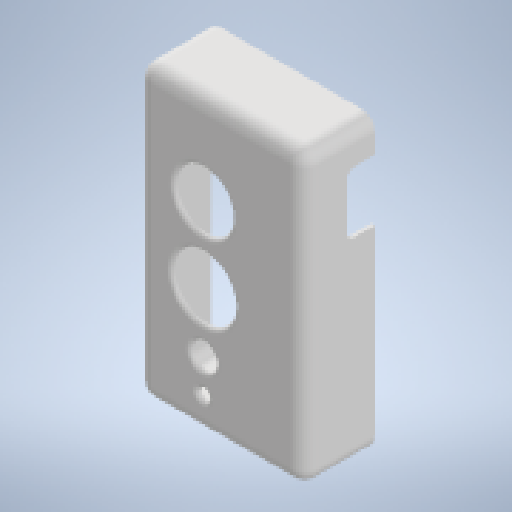
# Autodesk Inventor part: Part2
Saved by Autodesk Inventor 2025.2 (Build 292293000, 293)
## iProperties
Created: 2026-02-22
Part Number: Part2
Material: 一般
Document SubType Name: Modeling
Designer: naka6
Density: 1 g/cm^3
Appearance: 既定
Author: naka6
Autodesk Inventor part; units mm, degrees
ref_plane "YZ Plane" through (0, 0, 0) normal (1, 0, 0) x (0, 1, 0)
ref_plane "XZ Plane" through (0, 0, 0) normal (0, 1, 0) x (-1, 0, 0)
ref_plane "XY Plane" through (0, 0, 0) normal (0, 0, 1) x (1, 0, 0)
sketch "スケッチ1" plane through (0, 0, 0) normal (0, 0, 1) x (1, 0, 0)
  line L0 (17.8, -27.8) -> (17.8, 27.8) projected
  arc A0 (17.8, 27.8) -> (14.8, 30.8) centre (14.8, 27.8) ccw projected
  line L1 (14.8, 30.8) -> (-14.8, 30.8) projected
  arc A1 (-14.8, 30.8) -> (-17.8, 27.8) centre (-14.8, 27.8) ccw projected
  line L2 (-17.8, 27.8) -> (-17.8, -27.8) projected
  arc A2 (-17.8, -27.8) -> (-14.8, -30.8) centre (-14.8, -27.8) ccw projected
  line L3 (-14.8, -30.8) -> (14.8, -30.8) projected
  arc A3 (14.8, -30.8) -> (17.8, -27.8) centre (14.8, -27.8) ccw projected
  point P0 (0, 0)
extrude "押し出し1" add sketch "スケッチ1" along normal blind 15
fillet "フィレット1" radius 3 8 edges at (-16.9213, 29.9213, 15) (-17.8, 0, 15) (-16.9213, -29.9213, 15) (0, -30.8, 15) (16.9213, -29.9213, 15) (17.8, 0, 15) (16.9213, 29.9213, 15) (0, 30.8, 15)
shell "シェル1" thickness 0.8 removed faces 1 at (5.9333, 9.2667, 0)
sketch "スケッチ2" plane through (17.8, -27.8, 0) normal (1, 0, 0) x (0, 0, -1)
  line L0 (0, 51.6) -> (-6, 51.6)
  line L1 (-6, 51.6) -> (-6, 38.6)
  line L2 (-6, 38.6) -> (0, 38.6)
  line L3 (0, 38.6) -> (0, 51.6)
  line L4 (0, 58.6) -> (-12, 58.6) projected
  line L5 (0, 0) -> (0, 55.6) projected
  point P0 (0, 27.8)
  dimension "d4" = 6
  dimension "d5" = 7
  dimension "d6" = 20
  constraints: 8 end point, 2 parallel, 1 horizontal, 1 perpendicular, 1 point on line
  measures "d4" distance of L2.end L1.end
  measures "d5" distance between parallel lines of L0 L4
  measures "d6" distance between parallel lines of L4 L2
extrude "押し出し2" cut sketch "スケッチ2" against normal blind 15
fillet "フィレット2" radius 1.5 2 edges at (17.4, 10.8, 6) (17.4, 23.8, 6)
sketch "スケッチ3" plane through (0, 0, 15) normal (0, 0, 1) x (1, 0, 0)
  line L0 (-17.8, 27.8) -> (-17.8, -27.8) projected
  line L1 (-14.8, -30.8) -> (14.8, -30.8) projected
  line L2 (17.8, -27.8) -> (17.8, 27.8) projected
  line L3 (14.8, 30.8) -> (-14.8, 30.8) projected
  circle A0 centre (-3.8, 11.8) radius 6.15
  circle A1 centre (-3.8, -16.8) radius 2.65
  circle A2 centre (-3.8, -4.2) radius 6.65
  circle A3 centre (-3.8, -23.8) radius 1.15
  point P0 (0, 0)
  dimension "d10" = 12.3
  dimension "d11" = 19
  dimension "d12" = 14
  dimension "d14" = 5.3
  dimension "d15" = 13.3
  dimension "d16" = 2.3
  dimension "d17" = 14
  dimension "d18" = 14
  dimension "d19" = 7
  dimension "d20" = 14
  dimension "d21" = 14
  dimension "d22" = 35
  constraints: 4 centre point
  measures "d10" diameter of A0
  measures "d11" distance from line of L3 A0.centre
  measures "d12" distance from line of L0 A0.centre
  measures "d14" diameter of A1
  measures "d15" diameter of A2
  measures "d16" diameter of A3
  measures "d17" distance from line of L0 A3.centre
  measures "d18" distance from line of L0 A1.centre
  measures "d19" distance from line of L1 A3.centre
  measures "d20" distance from line of L1 A1.centre
  measures "d21" distance from line of L0 A2.centre
  measures "d22" distance from line of L3 A2.centre
extrude "押し出し3" cut sketch "スケッチ3" against normal blind 15
fillet "フィレット3" radius 1 4 edges at (-4.95, -23.8, 15) (-6.45, -16.8, 15) (-10.45, -4.2, 15) (-9.95, 11.8, 15)
